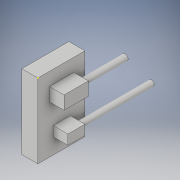
# Autodesk Inventor part: niharika1
Saved by Autodesk Inventor 2019 (Build 230136000, 136)
## iProperties
Created: 2020-02-13
Part Number: niharika1
Material: Generic
Document SubType Name: Modeling
Designer: Lenovo
Density: 1 g/cm^3
Appearance: Default
Author: Lenovo
Autodesk Inventor part; units mm, degrees
ref_plane "YZ Plane" through (0, 0, 0) normal (1, 0, 0) x (0, 1, 0)
ref_plane "XZ Plane" through (0, 0, 0) normal (0, 1, 0) x (-1, 0, 0)
ref_plane "XY Plane" through (0, 0, 0) normal (0, 0, 1) x (1, 0, 0)
sketch "Sketch1" plane through (0, 0, 0) normal (0, 1, 0) x (-1, 0, 0)
  line L0 (0, 0) -> (5.4973, 0)
  line L1 (5.4973, 0) -> (5.4973, -16.0791)
  line L2 (5.4973, -16.0791) -> (0, -16.0791)
  line L3 (0, -16.0791) -> (0, 0)
  constraints: 8 end point, 2 parallel, 1 horizontal, 1 perpendicular
extrude "Extrusion1" add sketch "Sketch1" along normal blind 25.4
sketch "Sketch2" plane through (0, 0, 0) normal (1, 0, 0) x (0, 0, -1)
  line L0 (5.242, 8.6906) -> (11.0751, 8.6906)
  line L1 (11.0751, 8.6906) -> (11.0751, 5.3799)
  line L2 (11.0751, 5.3799) -> (5.242, 5.3799)
  line L3 (5.242, 5.3799) -> (5.242, 8.6906)
  line L4 (12.2594, 20.9027) -> (3.9371, 20.9027)
  line L5 (3.9371, 20.9027) -> (3.9371, 16.3797)
  line L6 (3.9371, 16.3797) -> (12.2594, 16.3797)
  line L7 (12.2594, 16.3797) -> (12.2594, 20.9027)
  point P0 (0, 0)
  constraints: 16 end point, 4 parallel, 2 horizontal, 2 perpendicular
extrude "Extrusion2" add sketch "Sketch2" along normal blind 5
sketch "Sketch3" plane through (0, 25.4, 0) normal (0, 1, 0) x (1, 0, 0)
  point P0 (0, 0)
sketch "Sketch4" plane through (0, 16.3797, -12.2594) normal (0, 0, -1) x (-1, 0, 0)
  circle A0 centre (-2.546, 2.7504) radius 1.0051
  circle A1 centre (-2.546, -8.9893) radius 0.8063
  point P0 (0, -16.3797)
  constraints: 2 centre point
extrude "Extrusion3" add sketch "Sketch4" along normal blind 15 contours A0
sketch "Sketch5" plane through (0, 5.3799, -11.0751) normal (0, 0, -1) x (-1, 0, 0)
  circle A0 centre (-2.6874, 1.7983) radius 0.9619
  point P0 (0, -5.3799)
  constraints: 1 centre point
extrude "Extrusion4" add sketch "Sketch5" along normal blind 25
body "Solid1"
